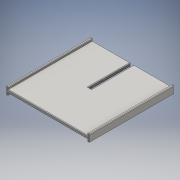
# Autodesk Inventor part: partition
Saved by Autodesk Inventor 2016 (Build 200138000, 138)
## iProperties
Created: 2017-04-06
Part Number: partition
Material: 一般
Document SubType Name: Modeling
Designer: Daisuke
Density: 1 g/cm^3
Appearance: 既定
Author: Daisuke
## iProperties of the stored document partition_3D プリント.ipt
Created: 2017-04-06
Part Number: partition_3D プリント
Material: 一般
Document SubType Name: Modeling
Designer: Daisuke
Density: 1 g/cm^3
Appearance: 既定
Author: Daisuke
Autodesk Inventor part; units mm, degrees
ref_plane "YZ Plane" through (0, 0, 0) normal (1, 0, 0) x (0, 1, 0)
ref_plane "XZ Plane" through (0, 0, 0) normal (0, 1, 0) x (-1, 0, 0)
ref_plane "XY Plane" through (0, 0, 0) normal (0, 0, 1) x (1, 0, 0)
sketch "スケッチ1" plane through (0, 0, 0) normal (0, 1, 0) x (-1, 0, 0)
  line L0 (37.5, 1.5) -> (-37.5, 1.5)
  line L1 (-37.5, 1.5) -> (-37.5, -1.5)
  line L2 (-37.5, -1.5) -> (37.5, -1.5)
  line L3 (37.5, -1.5) -> (37.5, 1.5)
  line L4 (37.5, 1.5) -> (-37.5, -1.5) construction
  line L5 (-37.5, 1.5) -> (37.5, -1.5) construction
  line L6 (36.5, 3.5) -> (38.5, 3.5)
  line L7 (38.5, 3.5) -> (38.5, -3.5)
  line L8 (38.5, -3.5) -> (36.5, -3.5)
  line L9 (36.5, -3.5) -> (36.5, 3.5)
  line L10 (36.5, 3.5) -> (38.5, -3.5) construction
  line L11 (38.5, 3.5) -> (36.5, -3.5) construction
  line L12 (-36.5, 3.5) -> (-38.5, 3.5)
  line L13 (-38.5, 3.5) -> (-38.5, -3.5)
  line L14 (-38.5, -3.5) -> (-36.5, -3.5)
  line L15 (-36.5, -3.5) -> (-36.5, 3.5)
  line L16 (-36.5, 3.5) -> (-38.5, -3.5) construction
  line L17 (-38.5, 3.5) -> (-36.5, -3.5) construction
  point P0 (0, 0)
  point P1 (37.5, 0)
  point P2 (-37.5, 0)
  dimension "d0" = 75
  dimension "d1" = 3
  dimension "d2" = 2
  dimension "d3" = 7
  dimension "d4" = 2
  dimension "d5" = 7
  constraints: 36 end point, 8 midpoint, 6 parallel, 3 horizontal, 3 perpendicular
  measures "d0" distance of L2.end L1.end
  measures "d1" distance of L1.end L0.end
  measures "d2" distance of L7.end L8.end
  measures "d3" distance of L6.end L7.end
  measures "d4" distance of L14.end L13.end
  measures "d5" distance of L13.end L12.end
extrude "押し出し1" add sketch "スケッチ1" along normal blind 78
sketch "スケッチ2" plane through (0, 78, 0) normal (0, 1, 0) x (1, 0, 0)
  line L0 (1.55, -1.5) -> (-1.55, -1.5)
  line L1 (-1.55, -1.5) -> (-1.55, 1.5)
  line L2 (-1.55, 1.5) -> (1.55, 1.5)
  line L3 (1.55, 1.5) -> (1.55, -1.5)
  line L4 (1.55, -1.5) -> (-1.55, 1.5) construction
  line L5 (-1.55, -1.5) -> (1.55, 1.5) construction
  point P0 (0, 0)
  dimension "d8" = 3.1
  dimension "d9" = 3
  constraints: 12 end point, 2 midpoint, 2 parallel, 1 horizontal, 1 perpendicular
  measures "d8" distance of L1.end L2.end
  measures "d9" distance of L0.end L1.end
extrude "押し出し2" cut sketch "スケッチ2" against normal blind 39
fillet "フィレット1" radius 0.5 33 edges at (19.025, 78, -1.5) (19.025, 78, 1.5) (1.55, 78, 0) (1.55, 58.5, 1.5) (1.55, 58.5, -1.5) (-1.55, 58.5, -1.5) (0, 39, -1.5) (0, 39, 1.5) (-1.55, 58.5, 1.5) (-1.55, 78, 0) (-19.025, 78, 1.5) (-19.025, 78, -1.5) (36.5, 78, 2.5) (37.5, 78, 3.5) (38.5, 78, 0) (37.5, 78, -3.5) (36.5, 78, -2.5) (36.5, 39, -3.5) (38.5, 39, -3.5) (38.5, 39, 3.5) (36.5, 39, 3.5) (-36.5, 39, 3.5) (-37.5, 78, 3.5) (-36.5, 78, 2.5) (-38.5, 78, 0) (-36.5, 78, -2.5) (-37.5, 78, -3.5) (-36.5, 39, -3.5) (-38.5, 39, -3.5) (-38.5, 39, 3.5) (-38.5, 0, 0) (-37.5, 0, 3.5) (-36.5, 0, 2.5)
fillet "フィレット2" radius 0.5 20 edges at (-36.75, 0, 1.5) (0, 0, 1.5) (0, 0, -1.5) (-37, 0, -2.25) (-37, 0, 2.25) (-37.5, 0, 3) (36.6464, 0, 3.3536) (-38, 0, 0) (-37.5, 0, -3) (38.3536, 0, 3.3536) (38.3536, 0, -3.3536) (36.6462, 0, -3.3538) (-38.3536, 0.1464, 3) (-38.5, 0.5, 0) (-38.3536, 0.1464, -3) (37.5, 0, 3.5) (38.5, 0, 0) (37.4995, 0, -3.5) (36.5, 0, -2.2505) (36.5, 0, 2.25)
